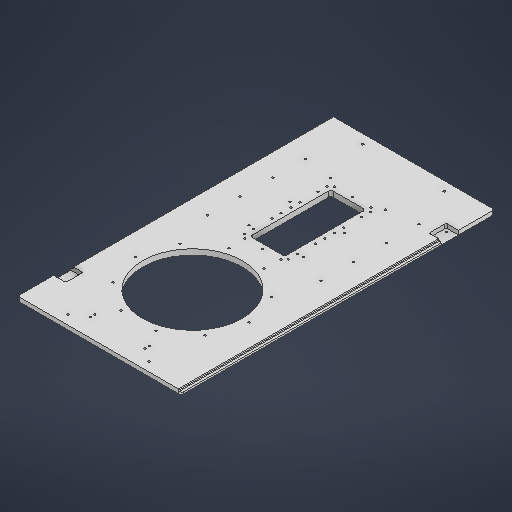
# Autodesk Inventor part: Updated Cover (Vibrometer)
Saved by Autodesk Inventor 2025 (Build 290162000, 162)
## iProperties
Created: 2024-04-25
Part Number: Updated Cover (Vibrometer)
Material: Generic
Document SubType Name: Modeling
Designer: Thienan Hoang
Density: 1 g/cm^3
Appearance: Default
Author: Thienan Hoang
Autodesk Inventor part; units mm, degrees
ref_plane "YZ Plane" through (0, 0, 0) normal (1, 0, 0) x (0, 1, 0)
sketch "Sketch1" plane through (0, 0, 0) normal (0, 1, 0) x (-1, 0, 0)
  line L0 (180, 345) -> (-180, 345)
  line L1 (-180, 345) -> (-180, -345)
  line L2 (-180, -345) -> (180, -345)
  line L3 (180, -345) -> (180, 345)
  line L4 (180, 345) -> (-180, -345) construction
  line L5 (-180, 345) -> (180, -345) construction
  point P0 (0, 0)
  dimension "d0" = 360
  dimension "d1" = 690
  constraints: 12 end point, 2 midpoint, 2 parallel, 1 horizontal, 1 perpendicular
  measures "d0" distance of L2.end L1.end
  measures "d1" distance of L1.end L0.end
extrude "Extrusion1" add sketch "Sketch1" along normal blind 12
sketch "Sketch2" plane through (0, 12, 0) normal (0, 1, 0) x (1, 0, 0)
  circle A0 centre (0, -140) radius 110
  line L0 (-180, -345) -> (180, -345) projected
  circle A1 centre (0, -140) radius 135
  point P0 (0, 0)
  dimension "d4" = 205
  dimension "d5" = 220
  dimension "d8" = 270
  constraints: 2 centre point, 1 coincident
  measures "d4" distance from line of A0.centre L0
  measures "d5" diameter of A0
  measures "d8" diameter of A1
extrude "Extrusion2" cut sketch "Sketch2" against normal through all contours A0
ref_plane "Work Plane1" through (0, 0, 150) normal (0, 0, 1) x (1, 0, 0)
sketch "Sketch6" plane through (0, 12, 0) normal (0, 1, 0) x (1, 0, 0)
  line L0 (89.6938, -325) -> (-89.6938, -325)
  line L1 (-89.6938, -325) -> (-89.6938, 325)
  line L2 (-89.6938, 325) -> (89.6938, 325)
  line L3 (89.6938, 325) -> (89.6938, -325)
  line L4 (89.6938, -325) -> (-89.6938, 325) construction
  line L5 (-89.6938, -325) -> (89.6938, 325) construction
  point P0 (0, 0)
  dimension "d55" = 179.3875
  dimension "d56" = 650
  constraints: 12 end point, 2 midpoint, 2 parallel, 1 horizontal, 1 perpendicular
  measures "d55" distance of L1.end L2.end
  measures "d56" distance of L0.end L1.end
hole "Hole3" at (89.6938, 12, 325) at (-89.6938, 12, 325) at (-89.6938, 12, -325) at (89.6938, 12, -325) direction (0, -1, 0) diameter 4.917 depth 10 tip angle 118 thread size "M6x1" class "6H" standard "ANSI Metric M Profile"
sketch "Sketch7" plane through (0, 12, 0) normal (0, 1, 0) x (1, 0, 0)
  circle A0 centre (0, -140) radius 110 projected
  circle A1 centre (0, -140) radius 131.5
  circle A2 centre (0, -140) radius 135
  point P0 (0, 0)
  dimension "d64" = 263
  dimension "d65" = 270
  constraints: 2 centre point, 2 coincident
  measures "d64" diameter of A1
  measures "d65" diameter of A2
ref_plane "Work Plane2" through (0, 15.875, 140) normal (0, 1, 0) x (1, 0, 0)
sketch "Sketch8" plane through (0, 15.875, 140) normal (0, 1, 0) x (1, 0, 0)
  circle A0 centre (0, 0) radius 131.5 projected
  circle A1 centre (0, 0) radius 125
  circle A2 centre (125, 0) radius 2
  circle A3 centre (101.1271, 73.4732) radius 2
  circle A4 centre (38.6271, 118.8821) radius 2
  circle A5 centre (-38.6271, 118.8821) radius 2
  circle A6 centre (-101.1271, 73.4732) radius 2
  circle A7 centre (-125, 0) radius 2
  circle A8 centre (-101.1271, -73.4732) radius 2
  circle A9 centre (-38.6271, -118.8821) radius 2
  circle A10 centre (38.6271, -118.8821) radius 2
  circle A11 centre (101.1271, -73.4732) radius 2
  point P0 (0, 140)
  dimension "d68" = 250
  dimension "d69" = 4
  dimension "d72" = 360
  constraints: 10 centre point, 1 coincident, 1 horizontal alignment, 23 other
  measures "d69" diameter of A2
hole "Hole4" at (125, 15.875, 140) at (101.1271, 15.875, 213.4732) at (38.6271, 15.875, 258.8821) at (-38.6271, 15.875, 258.8821) at (-101.1271, 15.875, 213.4732) at (-125, 15.875, 140) at (-101.1271, 15.875, 66.5268) at (-38.6271, 15.875, 21.1179) at (38.6271, 15.875, 21.1179) at (101.1271, 15.875, 66.5268) direction (0, -1, 0) diameter 4.134 depth 10 tip angle 118 thread size "M5x0.8" class "6H" standard "ANSI Metric M Profile"
sketch "Sketch9" plane through (0, 12, 0) normal (0, 1, 0) x (1, 0, 0)
  line L0 (180, -345) -> (180, 345) projected
  line L1 (180, 266) -> (156, 266)
  line L2 (153, 263) -> (153, 231)
  line L3 (156, 228) -> (180, 228)
  line L4 (180, 228) -> (180, 266)
  line L5 (-180, 345) -> (-180, -345) projected
  line L6 (-180, -266) -> (-156, -266)
  line L7 (-153, -263) -> (-153, -231)
  line L8 (-156, -228) -> (-180, -228)
  line L9 (-180, -228) -> (-180, -266)
  line L10 (180, 345) -> (-180, 345) projected
  line L11 (-180, -345) -> (180, -345) projected
  arc A0 (153, 231) -> (156, 228) centre (156, 231) ccw
  arc A1 (156, 266) -> (153, 263) centre (156, 263) ccw
  arc A2 (-156, -266) -> (-153, -263) centre (-156, -263) ccw
  arc A3 (-153, -231) -> (-156, -228) centre (-156, -231) ccw
  point P0 (0, 0)
  point P1 (153, 228)
  point P2 (153, 266)
  point P3 (-153, -228)
  point P4 (-153, -266)
  dimension "d82" = 27
  dimension "d83" = 27
  dimension "d84" = 38
  dimension "d85" = 38
  dimension "d86" = 79
  dimension "d87" = 79
  dimension "d95" = 3
  dimension "d96" = 3
  constraints: 16 end point, 10 point on line, 8 point on circle, 8 tangent, 4 centre point, 4 parallel, 2 equal radius, 2 horizontal, 2 perpendicular
  measures "d82" distance of L1.start point (153, 266)
  measures "d83" distance of point (-153, -228) L8.end
  measures "d84" distance of point (-153, -266) point (-153, -228)
  measures "d85" distance of point (153, 266) point (153, 228)
  measures "d86" distance between parallel lines of L10 L1
  measures "d87" distance between parallel lines of L11 L6
  measures "d95" radius of A0
  measures "d96" radius of A1
fillet "Fillet2" radius 5 2 edges at (180, 6, -345) (-180, 6, 345)
extrude "Extrusion7" cut sketch "Sketch9" against normal blind 9 contours L3 A0 L2 A1 L1 L0 | L5 L8 A3 L7 A2 L6
sketch "Sketch10" plane through (0, 12, 0) normal (0, 1, 0) x (1, 0, 0)
  line L0 (175, 345) -> (-180, 345) projected
  line L1 (-180, -228) -> (-174, -228)
  line L2 (-174, -228) -> (-174, 345)
  line L3 (-174, 345) -> (-180, 345)
  line L4 (-180, 345) -> (-180, -228)
  line L5 (180, 228) -> (156, 228) projected
  line L6 (-175, -345) -> (180, -345) projected
  line L7 (180, 228) -> (174, 228)
  line L8 (174, 228) -> (174, -345)
  line L9 (174, -345) -> (180, -345)
  line L10 (180, -345) -> (180, 228)
  point P0 (0, 0)
  point P1 (180, -345)
  point P2 (179.925, 228)
  dimension "d99" = 6
  dimension "d100" = 6
  constraints: 16 end point, 4 parallel, 2 horizontal, 2 perpendicular, 2 point on line
  measures "d99" distance of L3.end L2.end
  measures "d100" distance of L9.end L8.end
extrude "Extrusion8" cut sketch "Sketch10" against normal blind 3.1
chamfer "Chamfer3" distance 2 distance2 3.5 1 edges at (180, 8.9, 58.5) measured on face at (180, 3.9667, 154)
chamfer "Chamfer4" distance 2 distance2 3.5 1 edges at (-180, 8.9, -58.5) measured on face at (-180, 3.9667, -154)
sketch "Sketch11" plane through (0, 3, 0) normal (0, 1, 0) x (1, 0, 0)
  circle A0 centre (-161, -236) radius 1.65
  circle A1 centre (-161, -258) radius 1.65
  circle A2 centre (161, 258) radius 1.65
  circle A3 centre (161, 236) radius 1.65
  line L0 (-156, -266) -> (-180, -266) projected
  line L1 (174, 228) -> (156, 228) projected
  point P0 (0, 0)
  dimension "d110" = 8
  dimension "d111" = 22
  dimension "d113" = 3.3
  dimension "d114" = 3.3
  dimension "d115" = 3.3
  dimension "d116" = 3.3
  dimension "d118" = 8
  dimension "d119" = 22
  constraints: 4 centre point
  measures "d110" distance from line of L0 A1.centre
  measures "d111" distance of A1.centre A0.centre
  measures "d113" diameter of A0
  measures "d114" diameter of A1
  measures "d115" diameter of A3
  measures "d116" diameter of A2
  measures "d118" distance from line of L1 A3.centre
  measures "d119" distance of A3.centre A2.centre
hole "Hole5" at (-161, 3, 258) at (-161, 3, 236) at (161, 3, -236) at (161, 3, -258) direction (0, -1, 0) diameter 3.242 end through all thread size "M4x0.7" class "6H" standard "ANSI Metric M Profile"
chamfer "Chamfer5" distance 0.35 angle 45 4 edges at (-161, 3, 256.379) (-161, 3, 234.379) (161, 3, -259.621) (161, 3, -237.621)
sketch "Sketch12" plane through (0, 12, 0) normal (0, 1, 0) x (1, 0, 0)
  line L0 (50.125, 342.5) -> (-50.125, 342.5)
  line L1 (-50.125, 342.5) -> (-50.125, -342.5)
  line L2 (-50.125, -342.5) -> (50.125, -342.5)
  line L3 (50.125, -342.5) -> (50.125, 342.5)
  line L4 (50.125, 342.5) -> (-50.125, -342.5) construction
  line L5 (-50.125, 342.5) -> (50.125, -342.5) construction
  line L6 (-70.125, -362.5) -> (-70.125, 362.5)
  line L7 (-70.125, 362.5) -> (70.125, 362.5)
  line L8 (70.125, 362.5) -> (70.125, -362.5)
  line L9 (70.125, -362.5) -> (-70.125, -362.5)
  line L10 (-60.125, -352.5) -> (-60.125, 352.5)
  line L11 (-60.125, 352.5) -> (60.125, 352.5)
  line L12 (60.125, 352.5) -> (60.125, -352.5)
  line L13 (60.125, -352.5) -> (-60.125, -352.5)
  circle A0 centre (-60.125, 315) radius 2
  circle A1 centre (-60.125, 285) radius 2
  circle A2 centre (-60.125, 255) radius 2
  circle A3 centre (-60.125, 225) radius 2
  circle A4 centre (-60.125, 195) radius 2
  circle A5 centre (-60.125, 165) radius 2
  circle A6 centre (-60.125, 135) radius 2
  circle A7 centre (-60.125, 105) radius 2
  circle A8 centre (-60.125, 75) radius 2
  circle A9 centre (-60.125, 45) radius 2
  circle A10 centre (-60.125, -325) radius 2
  circle A11 centre (-60.125, -305) radius 2
  circle A12 centre (-60.125, -285) radius 2
  line L14 (0, 362.5) -> (0, -362.5)
  circle A13 centre (60.125, 315) radius 2
  circle A14 centre (60.125, 285) radius 2
  circle A15 centre (60.125, 255) radius 2
  circle A16 centre (60.125, 225) radius 2
  circle A17 centre (60.125, 195) radius 2
  circle A18 centre (60.125, 165) radius 2
  circle A19 centre (60.125, 135) radius 2
  circle A20 centre (60.125, 105) radius 2
  circle A21 centre (60.125, 75) radius 2
  circle A22 centre (60.125, 45) radius 2
  circle A23 centre (60.125, -325) radius 2
  circle A24 centre (60.125, -305) radius 2
  circle A25 centre (60.125, -285) radius 2
  line L15 (-125, 346.075) -> (125, 346.075)
  line L16 (125, 346.075) -> (125, -346.075)
  line L17 (125, -346.075) -> (-125, -346.075)
  line L18 (-125, -346.075) -> (-125, 346.075)
  line L19 (-125, 346.075) -> (125, -346.075) construction
  line L20 (125, 346.075) -> (-125, -346.075) construction
  circle A26 centre (-125, 270) radius 2
  line L21 (175, 345) -> (-174, 345) projected
  circle A27 centre (-125, 234) radius 2
  circle A28 centre (-125, 198) radius 2
  circle A29 centre (-125, 162) radius 2
  circle A30 centre (125, 270) radius 2
  circle A31 centre (125, 234) radius 2
  circle A32 centre (125, 198) radius 2
  circle A33 centre (125, 162) radius 2
  circle A34 centre (-125, 126) radius 2
  circle A35 centre (-125, 90) radius 2
  circle A36 centre (-125, 54) radius 2
  circle A37 centre (-125, 18) radius 2
  circle A38 centre (125, 126) radius 2
  circle A39 centre (125, 90) radius 2
  circle A40 centre (125, 54) radius 2
  circle A41 centre (125, 18) radius 2
  circle A42 centre (-60.125, -295.275) radius 2
  circle A43 centre (60.125, -295.275) radius 2
  point P0 (0, 0)
  dimension "d146" = 100.25
  dimension "d147" = 20
  dimension "d148" = 10
  dimension "d149" = 4
  dimension "d152" = 30
  dimension "d157" = 4
  dimension "d160" = 20
  dimension "d165" = 250
  dimension "d166" = 4
  dimension "d167" = 75
  dimension "d168" = 30
  dimension "d171" = 36
  dimension "d236" = 4
  dimension "d237" = 4
  constraints: 44 centre point, 42 end point, 21 symmetric about line, 8 parallel, 6 midpoint, 5 point on line, 4 perpendicular, 3 vertical, 2 horizontal, 63 other
  measures "d146" distance of L2.end L1.end
  measures "d147" distance between parallel lines of L1 L6
  measures "d148" distance between parallel lines of L1 L10
  measures "d149" diameter of A0
  measures "d152" distance of A0.centre A1.centre
  measures "d157" diameter of A10
  measures "d160" distance of A10.centre A11.centre
  measures "d165" distance of L16.end L17.end
  measures "d166" diameter of A26
  measures "d167" distance from line of L21 A26.centre
  measures "d168" distance from line of L21 A0.centre
  measures "d171" distance of A26.centre A27.centre
  measures "d236" diameter of A42
  measures "d237" diameter of A43
hole "Hole6" at (-60.125, 12, 305) at (60.125, 12, 305) at (-60.125, 12, -135) at (-60.125, 12, -225) at (60.125, 12, -225) at (60.125, 12, -135) at (-125, 12, -234) at (-125, 12, -162) at (125, 12, -162) at (125, 12, -234) at (-60.125, 12, -45) at (60.125, 12, -45) at (-125, 12, -90) at (-125, 12, -18) at (125, 12, -90) at (125, 12, -18) at (-60.125, 12, 295.275) at (60.125, 12, 295.275) direction (0, -1, 0) diameter 4.134 depth 10 tip angle 118 thread size "M5x0.8" class "6H" standard "ANSI Metric M Profile"
sketch "Sketch15" plane through (0, 12, 0) normal (0, 1, 0) x (1, 0, 0)
  line L0 (-38.1, 202.8) -> (38.1, 202.8)
  line L1 (38.1, 202.8) -> (38.1, 25)
  line L2 (38.1, 25) -> (-38.1, 25)
  line L3 (-38.1, 25) -> (-38.1, 202.8)
  line L4 (-38.1, 202.8) -> (38.1, 25) construction
  line L5 (38.1, 202.8) -> (-38.1, 25) construction
  circle A0 centre (0, -140) radius 110 projected
  line L6 (-48.1, 212.8) -> (48.1, 212.8)
  line L7 (48.1, 212.8) -> (48.1, 15)
  line L8 (48.1, 15) -> (-48.1, 15)
  line L9 (-48.1, 15) -> (-48.1, 212.8)
  circle A1 centre (0, 15) radius 2.5
  circle A2 centre (-20, 15) radius 2.5
  circle A3 centre (20, 15) radius 2.5
  circle A4 centre (-40, 15) radius 2.5
  circle A5 centre (40, 15) radius 2.5
  circle A6 centre (-48.1, 23.1) radius 2.5
  line L10 (-48.1, 113.9) -> (48.1, 113.9)
  circle A7 centre (-48.1, 43.1) radius 2.5
  circle A8 centre (-48.1, 63.1) radius 2.5
  circle A9 centre (-48.1, 83.1) radius 2.5
  circle A10 centre (-48.1, 103.1) radius 2.5
  line L11 (0, 15) -> (0, 212.8)
  circle A11 centre (48.1, 23.1) radius 2.5
  circle A12 centre (48.1, 43.1) radius 2.5
  circle A13 centre (48.1, 63.1) radius 2.5
  circle A14 centre (48.1, 83.1) radius 2.5
  circle A15 centre (48.1, 103.1) radius 2.5
  circle A16 centre (0, 212.8) radius 2.5
  circle A17 centre (-20, 212.8) radius 2.5
  circle A18 centre (20, 212.8) radius 2.5
  circle A19 centre (-40, 212.8) radius 2.5
  circle A20 centre (40, 212.8) radius 2.5
  circle A21 centre (-48.1, 204.7) radius 2.5
  circle A22 centre (-48.1, 184.7) radius 2.5
  circle A23 centre (-48.1, 164.7) radius 2.5
  circle A24 centre (-48.1, 144.7) radius 2.5
  circle A25 centre (-48.1, 124.7) radius 2.5
  circle A26 centre (48.1, 204.7) radius 2.5
  circle A27 centre (48.1, 164.7) radius 2.5
  circle A28 centre (48.1, 144.7) radius 2.5
  circle A29 centre (48.1, 184.7) radius 2.5
  circle A30 centre (48.1, 124.7) radius 2.5
  point P0 (0, 0)
  point P1 (0, 113.9)
  point P2 (0, 25)
  dimension "d191" = 76.2
  dimension "d192" = 177.8
  dimension "d193" = 165
  dimension "d197" = 10
  dimension "d198" = 5
  dimension "d201" = 20
  dimension "d206" = 8.1
  dimension "d207" = 5
  dimension "d208" = 8.1
  dimension "d211" = 20
  constraints: 30 centre point, 24 end point, 19 symmetric about line, 7 midpoint, 4 parallel, 2 horizontal, 2 perpendicular, 1 point on line, 1 vertical, 39 other
  measures "d191" distance of L1.end L2.end
  measures "d192" distance of L0.end L1.end
  measures "d193" distance of A0.centre point (0, 25)
  measures "d197" distance between parallel lines of L3 L9
  measures "d198" diameter of A1
  measures "d201" distance of L11.start A2.centre
  measures "d206" distance of L8.end A4.centre
  measures "d207" diameter of A6
  measures "d208" distance of L8.end A6.centre
  measures "d211" distance of A6.centre A7.centre
extrude "Extrusion11" cut sketch "Sketch15" against normal blind 21.1125 contours L0 L11 L10 L3 | L0 L1 L10 L11 | L10 L11 L2 L3 | L10 L1 L2 L11
fillet "Fillet3" radius 5 4 edges at (-38.1, 6, -202.8) (38.1, 6, -202.8) (-38.1, 6, -25) (38.1, 6, -25)
hole "Hole7" at (-48.1, 12, -23.1) at (-48.1, 12, -43.1) at (-48.1, 12, -83.1) at (-48.1, 12, -103.1) at (-48.1, 12, -124.7) at (-48.1, 12, -144.7) at (-48.1, 12, -184.7) at (-48.1, 12, -204.7) at (-40, 12, -212.8) at (0, 12, -212.8) at (40, 12, -212.8) at (48.1, 12, -204.7) at (48.1, 12, -184.7) at (48.1, 12, -144.7) at (48.1, 12, -124.7) at (48.1, 12, -103.1) at (48.1, 12, -83.1) at (48.1, 12, -43.1) at (48.1, 12, -23.1) at (40, 12, -15) at (0, 12, -15) at (-40, 12, -15) direction (0, -1, 0) diameter 4.134 depth 10 tip angle 118 thread size "M5x0.8" class "6H" standard "ANSI Metric M Profile"
fillet "Fillet5" radius 5 2 edges at (-180, 3.45, -345) (180, 3.45, 345)
chamfer "Chamfer6" distance 3 angle 45 8 edges at (180, 0, 0) (178.5355, 0, -343.5355) (0, 0, -345) (-178.5355, 0, -343.5355) (-180, 0, 0) (-178.5355, 0, 343.5355) (0, 0, 345) (178.5355, 0, 343.5355)
body "Solid1"
